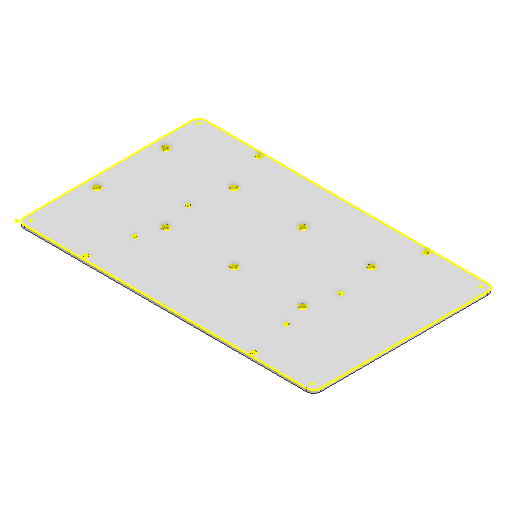
# Autodesk Inventor part: amplifier_tray
Saved by Autodesk Inventor 2023 (Build 270158000, 158)
## iProperties
Created: 2024-05-05
Part Number: amplifier_tray
Material: Generic
Document SubType Name: Modeling
Designer: Thomas
Density: 1 g/cm^3
Appearance: Default
Author: Thomas
Autodesk Inventor part; units mm, degrees
ref_plane "YZ Plane" through (0, 0, 0) normal (1, 0, 0) x (0, 1, 0)
ref_plane "XZ Plane" through (0, 0, 0) normal (0, 1, 0) x (-1, 0, 0)
ref_plane "XY Plane" through (0, 0, 0) normal (0, 0, 1) x (1, 0, 0)
sketch "Sketch1" plane through (0, 0, 0) normal (0, 1, 0) x (-1, 0, 0)
  line L0 (0, 0) -> (-215.9, 0)
  line L1 (-215.9, 0) -> (-215.9, -132.08)
  line L2 (-215.9, -132.08) -> (0, -132.08)
  line L3 (0, -132.08) -> (0, 0)
  circle A0 centre (-46.99, -129.008) radius 1.65
  circle A1 centre (-168.91, -129.008) radius 1.65
  circle A2 centre (-46.99, -3.072) radius 1.65
  circle A3 centre (-168.91, -3.072) radius 1.65
  circle A4 centre (-8, -50) radius 2.2
  circle A5 centre (-8, -100) radius 2.2
  circle A6 centre (-58, -50) radius 2.2
  circle A7 centre (-58, -100) radius 2.2
  circle A8 centre (-108, -50) radius 2.2
  circle A9 centre (-108, -100) radius 2.2
  circle A10 centre (-158, -50) radius 2.2
  circle A11 centre (-158, -100) radius 2.2
  circle A12 centre (-52.45, -72.08) radius 1.25
  circle A13 centre (-163.45, -72.08) radius 1.25
  circle A14 centre (-52.45, -33.08) radius 1.25
  circle A15 centre (-163.45, -33.08) radius 1.25
  dimension "d0" = 215.9
  dimension "d1" = 132.08
  dimension "d2" = 3.3
  dimension "d5" = 121.92
  dimension "d8" = 125.936
  dimension "d11" = 46.99
  dimension "d12" = 3.072
  dimension "d13" = 3.072
  dimension "d14" = 4.4
  dimension "d15" = 50
  dimension "d16" = 8
  dimension "d19" = 50
  dimension "d22" = 50
  dimension "d30" = 2.5
  dimension "d33" = 111
  dimension "d36" = 39
  dimension "d39" = 60
  dimension "d40" = 52.45
  constraints: 16 centre point, 8 end point, 4 horizontal, 3 vertical, 2 parallel, 1 perpendicular, 26 other
  measures "d0" distance of L1.end L2.end
  measures "d1" distance of L0.end L1.end
  measures "d2" diameter of A0
  measures "d5" distance of A0.centre A1.centre
  measures "d8" distance of A0.centre A2.centre
  measures "d11" distance from line of L3 A0.centre
  measures "d12" distance from line of L2 A0.centre
  measures "d13" distance from line of L0 A2.centre
  measures "d14" diameter of A4
  measures "d15" distance from line of L0 A4.centre
  measures "d16" distance from line of L3 A4.centre
  measures "d19" distance of A4.centre A5.centre
  measures "d22" distance of A4.centre A6.centre
  measures "d30" diameter of A12
  measures "d33" distance of A12.centre A13.centre
  measures "d36" distance of A12.centre A14.centre
  measures "d39" distance from line of L2 A12.centre
  measures "d40" distance from line of A13.centre L1
extrude "Extrusion1" add sketch "Sketch1" against normal blind 2.54
sketch "Sketch2" plane through (0, 0, 0) normal (0, 1, 0) x (1, 0, 0)
  line L0 (108.9107, 44.2653) -> (116.6369, 44.2653) construction
  line L1 (116.6369, 44.2653) -> (116.6369, 41.0888) construction
  line L2 (116.6369, 41.0888) -> (108.9107, 41.0888) construction
  line L3 (108.9107, 41.0888) -> (108.9107, 44.2653) construction
  point P0 (0, 0)
  constraints: 2 other
extrude "Extrusion2" [suppressed]
fillet "Fillet1" radius 5 4 edges at (0, -1.27, 0) (215.9, -1.27, 0) (215.9, -1.27, -132.08) (0, -1.27, -132.08)
sketch "Sketch3" plane through (0, 0, 0) normal (0, 1, 0) x (1, 0, 0)
  arc A0 (5, 132.08) -> (0, 127.08) centre (5, 127.08) ccw projected
  line L0 (0, 127.08) -> (0, 5) projected
  arc A1 (0, 5) -> (5, 0) centre (5, 5) ccw projected
  line L1 (5, 0) -> (210.9, 0) projected
  arc A2 (210.9, 0) -> (215.9, 5) centre (210.9, 5) ccw projected
  line L2 (215.9, 5) -> (215.9, 127.08) projected
  arc A3 (215.9, 127.08) -> (210.9, 132.08) centre (210.9, 127.08) ccw projected
  line L3 (210.9, 132.08) -> (5, 132.08) projected
  circle A4 centre (163.45, 33.08) radius 1.25 projected
  circle A5 centre (163.45, 72.08) radius 1.25 projected
  circle A6 centre (158, 100) radius 2.2 projected
  circle A7 centre (108, 100) radius 2.2 projected
  circle A8 centre (58, 100) radius 2.2 projected
  circle A9 centre (58, 50) radius 2.2 projected
  circle A10 centre (8, 100) radius 2.2 projected
  circle A11 centre (8, 50) radius 2.2 projected
  circle A12 centre (168.91, 3.072) radius 1.65 projected
  circle A13 centre (46.99, 3.072) radius 1.65 projected
  circle A14 centre (168.91, 129.008) radius 1.65 projected
  circle A15 centre (46.99, 129.008) radius 1.65 projected
  circle A16 centre (108, 50) radius 2.2 projected
  circle A17 centre (158, 50) radius 2.2 projected
  circle A18 centre (52.45, 72.08) radius 1.25 projected
  circle A19 centre (52.45, 33.08) radius 1.25 projected
  point P0 (0, 0)
equation "\"d40\" = -0.5 * d33 + 0.5 * d0"
body "Solid1"
